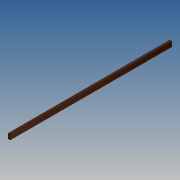
# Autodesk Inventor part: 2p3post
Saved by Autodesk Inventor 2014 SP1 (Build 180222100, 222)
## iProperties
Company: HERA Project
Created: 2013-06-11
Part Number: 2p3post
Material: Wood (Walnut)
Document SubType Name: Modeling
Designer: David DeBoer
Density: 0.55 g/cm^3
Description: Support stand post
Mass: 11457.8 g
Surface Area: 10259.2 cm^2
Volume: 20832.3 cm^3
Appearance: Walnut - Natural Polished
Author: David DeBoer
Title: Support stand post
Autodesk Inventor part; units mm, degrees
ref_plane "YZ Plane" through (0, 0, 0) normal (1, 0, 0) x (0, 1, 0)
ref_plane "XZ Plane" through (0, 0, 0) normal (0, 1, 0) x (-1, 0, 0)
ref_plane "XY Plane" through (0, 0, 0) normal (0, 0, 1) x (1, 0, 0)
sketch "Sketch1" plane through (0, 0, 0) normal (0, 0, 1) x (1, 0, 0)
  line L0 (0, 0) -> (50, 0)
  line L1 (50, 0) -> (50, 114)
  line L2 (50, 114) -> (0, 114)
  line L3 (0, 114) -> (0, 0)
  dimension "d0" = 50
  dimension "d1" = 114
  constraints: 8 end point, 2 parallel, 1 horizontal, 1 perpendicular
  measures "d0" distance of L0.start L0.end
  measures "d1" distance of L2.end L0.start
extrude "Extrusion1" add sketch "Sketch1" along normal blind 3657.6
sketch "Sketch4" plane through (0, 0, 3657.6) normal (0, 0, 1) x (1, 0, 0)
  circle A0 centre (25, 57) radius 12.7
  line L0 (0, 0) -> (50, 0) projected
  line L1 (50, 0) -> (50, 114) projected
  line L2 (50, 114) -> (0, 114) projected
  line L3 (0, 114) -> (0, 0) projected
  line L4 (25, 114) -> (25, 0) construction
  line L5 (0, 57) -> (50, 57) construction
  point P0 (25, 57)
  dimension "d16" = 25.4
  constraints: 5 midpoint, 4 end point, 1 centre point, 1 coincident
  measures "d16" diameter of A0
extrude "Extrusion4" cut sketch "Sketch4" against normal blind 254 contours A0
body "Solid1"
